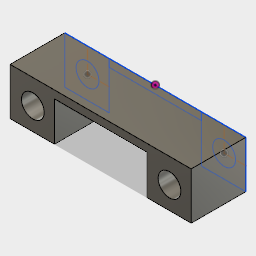
Feiyu Gimbal Mount Standin v2 (Autodesk Fusion 360 design; units mm, degrees)
Autodesk Fusion 360 part; units mm, degrees
sketch "Sketch1" plane through (0, 0, 0) normal (0, 0, 1) x (1, 0, 0)
  line L0 (-5.06, 0) -> (-9.94, 0)
  line L1 (-9.94, 0) -> (-9.94, -5.17)
  line L2 (-9.94, -5.17) -> (-5.06, -5.17)
  line L3 (-5.06, -5.17) -> (-5.06, 0)
  line L4 (-9.94, 0) -> (5.06, 0)
  line L5 (5.06, 0) -> (9.94, 0)
  line L6 (9.94, 0) -> (9.94, -5.17)
  line L7 (9.94, -5.17) -> (5.06, -5.17)
  line L8 (5.06, -5.17) -> (5.06, 0)
  line L9 (-5.06, 0) -> (5.06, 0)
  line L10 (5.06, 0) -> (5.06, -0.85)
  line L11 (5.06, -0.85) -> (-5.06, -0.85)
  line L12 (-5.06, -0.85) -> (-5.06, 0)
  circle A0 centre (7.56, -2.7) radius 1.25
  circle A1 centre (-7.44, -2.7) radius 1.25
  line L13 (-7.44, -2.7) -> (-5.06, -2.7) construction
  line L14 (-7.44, -2.7) -> (-7.44, 0) construction
  line L15 (7.56, -2.7) -> (7.56, 0) construction
  line L16 (7.56, -2.7) -> (9.94, -2.7) construction
  dimension "d1" = 4.88
  dimension "d2" = 5.17
  dimension "d4" = 0.85
  dimension "d5" = 2.5
  dimension "d6" = 2.7
  dimension "d7" = 2.5
  dimension "d10" = 15
  measures "d1" distance of L4.end L5.end
  measures "d2" distance of L5.end L6.end
  measures "d4" distance of L9 L11
  measures "d5" diameter of A0
  measures "d6" distance of L5 A0.centre
  measures "d7" distance of L8 A0.centre
  measures "d10" distance of A0.centre A1.centre
extrude "Extrude1" add sketch "Sketch1" along normal blind 6
